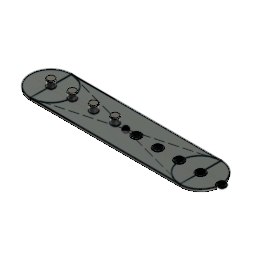
hat spacer v2 (Autodesk Fusion 360 design; units mm, degrees)
Autodesk Fusion 360 part; units mm, degrees
note: some values were not read from the file. Set by a fixed rule: which sketch regions a step uses.
sketch "Sketch1" plane through (0, 0, 0) normal (0, 0, 1) x (1, 0, 0)
  line L0 (30.17, 8.25) -> (-30.17, 8.25)
  line L1 (-30.17, 8.25) -> (-30.17, -8.25)
  line L2 (-30.17, -8.25) -> (30.17, -8.25)
  line L3 (30.17, -8.25) -> (30.17, 8.25)
  line L4 (30.17, 8.25) -> (-30.17, -8.25) construction
  line L5 (-30.17, 8.25) -> (30.17, -8.25) construction
  circle A0 centre (-30.17, 0) radius 8.25
  circle A1 centre (30.17, 0) radius 8.25
  circle A2 centre (-30.17, 0) radius 1.425
  circle A3 centre (-21.55, 0) radius 1.425
  circle A4 centre (-12.93, 0) radius 1.425
  circle A5 centre (-4.31, 0) radius 1.425
  circle A6 centre (4.31, 0) radius 1.425
  circle A7 centre (12.93, 0) radius 1.425
  circle A8 centre (21.55, 0) radius 1.425
  circle A9 centre (30.17, 0) radius 1.425
  circle A10 centre (38.79, 0) radius 1.425
  point P0 (-21.55, 0)
  point P1 (-12.93, 0)
  point P2 (-4.31, 0)
  point P3 (4.31, 0)
  point P4 (12.93, 0)
  point P5 (21.55, 0)
  point P6 (30.17, 0)
  point P7 (38.79, 0)
  dimension "d5" = 60.34
  dimension "d6" = 16.5
  dimension "d7" = 16.5
  dimension "d8" = 16.5
  dimension "d11" = 8.62
  dimension "d12" = 0
  dimension "d20" = 2.85
  constraint horizontal L0
  constraint perpendicular L0 L1
  constraint parallel L0 L2
  constraint parallel L1 L3
  constraint coincident L4 origin
  constraint coincident L5 origin
  constraint midpoint L1 A0.centre
  constraint midpoint L3 P6
  constraint concentric A0 A2
  measures "d5" distance of L1.end L2.end
  measures "d6" distance of L0.end L1.end
  measures "d7" diameter of A0
  measures "d8" diameter of A1
  measures "d20" diameter of A2
extrude "Extrude1" add sketch "Sketch1" against normal blind 1 contours L0 L2 A0 A1 A3 A8 | L3 A1 A9 A10 | L3 A1 A8 A9 | L1 A0 A2 A3 | L1 A0 A2 | L3 A9 | L3 A9 | A1 A10 | A1 A8 | A1 A8 | L1 A2 | L1 A2 | A0 A3 | A0 A3 | A4 | A5 | A6 | A7 picked at (38.0754, -0.2518)
hole "Hole1" at (30.17, 0, 0) at (21.55, 0, 0) at (12.93, 0, 0) at (4.31, 0, 0) at (38.79, 0, 0) direction (0, 0, -1) diameter 2.98 depth 1 tip angle 180 counterbore diameter 3.78 counterbore depth 0.1
extrude "Extrude2" add sketch "Sketch1" along normal blind 2.3 contours L1 A2 | L1 A2 | A0 A3 | A0 A3 | A4 | A5
extrude "Extrude3" add 4 faces at (-29.742, 0.2061, 2.3) (-21.1404, 0.7307, 2.3) (-12.4592, -0.4905, 2.3) (-5.0064, 0.28, 2.3) along direction (0, 0, 1) blind 0.5 draft 40
fillet "Fillet1" radius 0.2 4 edges at (-6.0297, 0.667, 2.8) (-14.6497, 0.667, 2.8) (-23.2697, 0.667, 2.8) (-31.8897, 0.667, 2.8)
equation "strapwidth = 16.5 mm"
equation "holedia = 2.98 mm"
equation "holespacing = 11.6 mm - holedia"
equation "pegdia = 2.85 mm"
equation "d5 = holespacing * 7"
equation "d6 = strapwidth"
equation "d7 = strapwidth"
equation "d8 = strapwidth"
equation "d11 = holespacing"
equation "d16 = holedia"
equation "d19 = holedia + 0.8 mm"
equation "d20 = pegdia"
named bodies: "hat adaptor"
